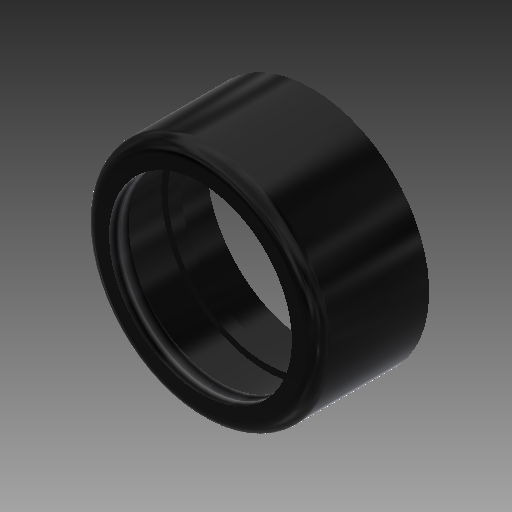
# Autodesk Inventor part: 201-02
Saved by Autodesk Inventor 2019 (Build 230136000, 136)
## iProperties
Company: Autodesk Inc
Created: 2017-06-27
Part Number: 201-02
Material: PC/ABS Plastic
Document SubType Name: Modeling
Designer: Autodesk Inc
Density: 0.357273 g/cm^3
Appearance: Smooth - Black
Mass: 1.5353 g
Surface Area: 44.8158 cm^2
Volume: 4.29727 cm^3
Author: Inventor
Autodesk Inventor part; units mm, degrees
ref_plane "YZ Plane" through (0, 0, 0) normal (1, 0, 0) x (0, 1, 0)
ref_plane "XZ Plane" through (0, 0, 0) normal (0, 1, 0) x (-1, 0, 0)
ref_plane "XY Plane" through (0, 0, 0) normal (0, 0, 1) x (1, 0, 0)
sketch "Sketch1" plane through (0, 0, 0) normal (1, 0, 0) x (0, 1, 0)
  line L0 (16, 0) -> (16, 5)
  line L1 (16, 5) -> (15, 5)
  line L2 (15, 5) -> (15, 7)
  line L3 (15, 7) -> (16, 7)
  line L4 (16, 7) -> (16, 14)
  line L5 (16, 14) -> (14, 14)
  line L6 (14, 14) -> (14, 17)
  line L7 (18, 0) -> (18, 17)
  line L8 (18, 17) -> (14, 17)
  line L9 (16, 0) -> (18, 0)
  line L10 (0, 0) -> (0, 15) construction
  dimension "d0" = 5
  dimension "d1" = 16
  dimension "d2" = 1
  dimension "d3" = 2
  dimension "d4" = 7
  dimension "d8" = 14
  dimension "d9" = 3
  dimension "d10" = 18
  constraints: 22 end point, 5 vertical, 3 horizontal, 2 horizontal alignment, 2 perpendicular, 1 parallel, 1 vertical alignment
  measures "d0" distance of L0.start L0.end
  measures "d1" distance of L10.start L0.start
  measures "d2" distance of L2.end L3.end
  measures "d3" distance of L1.end L2.end
  measures "d4" distance of L3.end L4.end
  measures "d8" horizontal distance of L10.start L5.end
  measures "d9" distance of L5.end L6.end
  measures "d10" distance of L10.start L7.start
revolve "Revolution1" add sketch "Sketch1" angle 360 about axis through (0, 0, 0) along (0, 0, 1)
thread "Thread1" size "M28x2" class "6H" standard "ANSI Metric M Profile" full length
fillet "Fillet1" radius 2 1 edges at (0, -18, 17)
body "Solid1"
